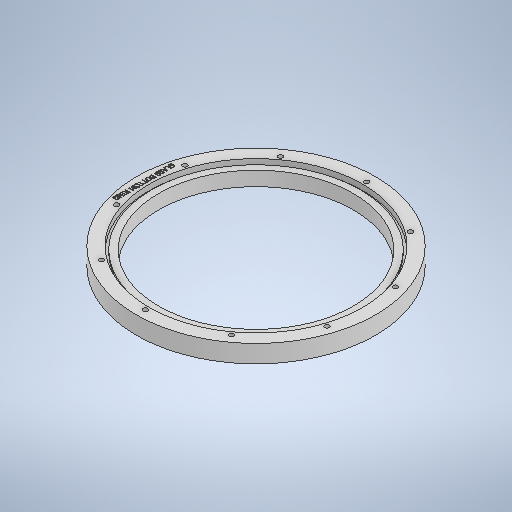
# Autodesk Inventor part: GlassBottomRing
Saved by Autodesk Inventor 2025 (Build 290162000, 162)
## iProperties
Created: 2025-06-19
Part Number: GlassBottomRing
Material: Generic
Document SubType Name: Modeling
Designer: mumin
Density: 1 g/cm^3
Appearance: Default
Author: mumin
Autodesk Inventor part; units mm, degrees
ref_plane "YZ Plane" through (0, 0, 0) normal (1, 0, 0) x (0, 1, 0)
ref_plane "XZ Plane" through (0, 0, 0) normal (0, 1, 0) x (-1, 0, 0)
ref_plane "XY Plane" through (0, 0, 0) normal (0, 0, 1) x (1, 0, 0)
sketch "Sketch1" plane through (0, 0, 0) normal (0, 1, 0) x (-1, 0, 0)
  circle A0 centre (0, 0) radius 110
  circle A1 centre (0, 0) radius 135
  dimension "d0" = 220
  dimension "d1" = 270
  constraints: 2 centre point, 2 coincident
  measures "d0" diameter of A0
  measures "d1" diameter of A1
extrude "Ring" add sketch "Sketch1" along normal blind 20
sketch "Sketch2" plane through (0, 20, 0) normal (0, 1, 0) x (1, 0, 0)
  circle A0 centre (0, 0) radius 120.5
  dimension "d4" = 241
  constraints: 1 centre point, 1 coincident
  measures "d4" diameter of A0
extrude "Glass Seat" cut sketch "Sketch2" against normal blind 3.9
sketch "Sketch3" plane through (0, 20, 0) normal (0, 1, 0) x (1, 0, 0)
  line L0 (0, 189) -> (0, -189) projected
  point P0 (0, 0)
  point P1 (0, 125)
  dimension "d14" = 125
  constraints: 1 point on line
  measures "d14" distance of point (0, 0) point (0, 125)
hole "Holes" at (0, 20, -125) direction (0, -1, 0) diameter 5.2 end through all
pattern_circular "Circular Pattern1" count 10 over 360 about axis through (0, -10, 0) along (0, 1, 0) of "Holes"
sketch "Sketch4" plane through (0, 20, 0) normal (0, 1, 0) x (1, 0, 0)
  line L0 (-123.4008, 33.078) -> (-123.4008, -40.8071) construction
  line L1 (-123.4008, -40.8071) -> (-126.5772, -40.8071) construction
  line L2 (-126.5772, -40.8071) -> (-126.5772, 33.078) construction
  line L3 (-126.5772, 33.078) -> (-123.4008, 33.078) construction
  spline S0 degree 2 poles (-128.6034, 30.4767) (-128.6034, 31.0075) (-128.2792, 31.8868) (-127.951, 32.2028) knots 0 0 0 1 2 2 2
  spline S1 degree 2 poles (-127.951, 32.2028) (-127.6188, 32.5189) (-126.6382, 32.8552) (-126.0021, 32.8552) knots 0 0 0 1 2 2 2
  spline S2 degree 2 poles (-126.0021, 32.8552) (-125.3984, 32.8552) (-124.4421, 32.5148) (-124.1018, 32.1988) knots 0 0 0 1 2 2 2
  spline S3 degree 2 poles (-124.1018, 32.1988) (-123.7736, 31.8949) (-123.417, 31.0035) (-123.417, 30.4727) knots 0 0 0 1 2 2 2
  spline S4 degree 2 poles (-123.417, 30.4727) (-123.417, 30.2174) (-123.4899, 29.7555) (-123.5548, 29.5448) knots 0 0 0 1 2 2 2
  spline S5 degree 2 poles (-123.5548, 29.5448) (-123.6034, 29.3746) (-123.7817, 28.9613) (-123.8465, 28.8357) knots 0 0 0 1 2 2 2
  line L4 (-123.8465, 28.8357) -> (-124.6488, 28.8357)
  line L5 (-124.6488, 28.8357) -> (-124.6488, 28.8925)
  spline S6 degree 2 poles (-124.6488, 28.8925) (-124.5394, 29.0181) (-124.3408, 29.2814) (-124.2274, 29.5245) knots 0 0 0 1 2 2 2
  spline S7 degree 2 poles (-124.2274, 29.5245) (-124.1261, 29.7271) (-123.9924, 30.2498) (-123.9924, 30.5497) knots 0 0 0 1 2 2 2
  spline S8 degree 2 poles (-123.9924, 30.5497) (-123.9924, 31.2709) (-125.0783, 32.1623) (-125.9818, 32.1623) knots 0 0 0 1 2 2 2
  spline S9 degree 2 poles (-125.9818, 32.1623) (-126.4843, 32.1623) (-127.2379, 31.9273) (-127.4972, 31.7044) knots 0 0 0 1 2 2 2
  spline S10 degree 2 poles (-127.4972, 31.7044) (-127.7566, 31.4897) (-128.028, 30.8819) (-128.028, 30.501) knots 0 0 0 1 2 2 2
  spline S11 degree 2 poles (-128.028, 30.501) (-128.028, 30.2215) (-127.947, 29.6623) (-127.866, 29.4719) knots 0 0 0 1 2 2 2
  line L6 (-127.866, 29.4719) -> (-126.5734, 29.4719)
  line L7 (-126.5734, 29.4719) -> (-126.5734, 30.6307)
  line L8 (-126.5734, 30.6307) -> (-125.9899, 30.6307)
  line L9 (-125.9899, 30.6307) -> (-125.9899, 28.8155)
  line L10 (-125.9899, 28.8155) -> (-128.1739, 28.8155)
  spline S12 degree 2 poles (-128.1739, 28.8155) (-128.2306, 28.9411) (-128.4048, 29.3706) (-128.4575, 29.5529) knots 0 0 0 1 2 2 2
  spline S13 degree 2 poles (-128.4575, 29.5529) (-128.5305, 29.8001) (-128.6034, 30.1972) (-128.6034, 30.4767) knots 0 0 0 1 2 2 2
  line L11 (-128.5061, 25.0837) -> (-128.5061, 27.9808)
  line L12 (-128.5061, 27.9808) -> (-123.5061, 27.9808)
  line L13 (-123.5061, 27.9808) -> (-123.5061, 27.3163)
  line L14 (-123.5061, 27.3163) -> (-127.9146, 27.3163)
  line L15 (-127.9146, 27.3163) -> (-127.9146, 25.0837)
  line L16 (-127.9146, 25.0837) -> (-128.5061, 25.0837)
  line L17 (-128.5061, 25.0999) -> (-123.5061, 23.4143)
  line L18 (-123.5061, 23.4143) -> (-123.5061, 22.5959)
  line L19 (-123.5061, 22.5959) -> (-128.5061, 20.9103)
  line L20 (-128.5061, 20.9103) -> (-128.5061, 21.6113)
  line L21 (-128.5061, 21.6113) -> (-127.1083, 22.0651)
  line L22 (-127.1083, 22.0651) -> (-127.1083, 23.9735)
  line L23 (-127.1083, 23.9735) -> (-128.5061, 24.4273)
  line L24 (-128.5061, 24.4273) -> (-128.5061, 25.0999)
  line L25 (-126.541, 22.2474) -> (-124.1869, 23.0213)
  line L26 (-124.1869, 23.0213) -> (-126.541, 23.7912)
  line L27 (-126.541, 23.7912) -> (-126.541, 22.2474)
  spline S14 degree 2 poles (-128.5953, 19.0424) (-128.5953, 19.5853) (-128.3684, 20.3471) (-128.2063, 20.6834) knots 0 0 0 1 2 2 2
  line L28 (-128.2063, 20.6834) -> (-127.3716, 20.6834)
  line L29 (-127.3716, 20.6834) -> (-127.3716, 20.6348)
  spline S15 degree 2 poles (-127.3716, 20.6348) (-127.6796, 20.3066) (-128.0199, 19.4759) (-128.0199, 19.091) knots 0 0 0 1 2 2 2
  spline S16 degree 2 poles (-128.0199, 19.091) (-128.0199, 18.5399) (-127.5621, 17.9767) (-127.1852, 17.9767) knots 0 0 0 1 2 2 2
  spline S17 degree 2 poles (-127.1852, 17.9767) (-126.8854, 17.9767) (-126.5126, 18.2725) (-126.4194, 18.5926) knots 0 0 0 1 2 2 2
  spline S18 degree 2 poles (-126.4194, 18.5926) (-126.3546, 18.8236) (-126.2655, 19.2085) (-126.1925, 19.4962) knots 0 0 0 1 2 2 2
  spline S19 degree 2 poles (-126.1925, 19.4962) (-126.1236, 19.7555) (-125.917, 20.1647) (-125.7509, 20.3228) knots 0 0 0 1 2 2 2
  spline S20 degree 2 poles (-125.7509, 20.3228) (-125.5848, 20.4767) (-125.139, 20.6469) (-124.8473, 20.6469) knots 0 0 0 1 2 2 2
  spline S21 degree 2 poles (-124.8473, 20.6469) (-124.2395, 20.6469) (-123.417, 19.6988) (-123.417, 18.9654) knots 0 0 0 1 2 2 2
  spline S22 degree 2 poles (-123.417, 18.9654) (-123.417, 18.544) (-123.5831, 17.7985) (-123.7412, 17.4784) knots 0 0 0 1 2 2 2
  line L30 (-123.7412, 17.4784) -> (-124.5353, 17.4784)
  line L31 (-124.5353, 17.4784) -> (-124.5353, 17.527)
  spline S23 degree 2 poles (-124.5353, 17.527) (-124.3165, 17.766) (-123.9924, 18.5116) (-123.9924, 18.9208) knots 0 0 0 1 2 2 2
  spline S24 degree 2 poles (-123.9924, 18.9208) (-123.9924, 19.3827) (-124.4259, 19.954) (-124.7784, 19.954) knots 0 0 0 1 2 2 2
  spline S25 degree 2 poles (-124.7784, 19.954) (-125.0945, 19.954) (-125.4713, 19.6177) (-125.5564, 19.3017) knots 0 0 0 1 2 2 2
  spline S26 degree 2 poles (-125.5564, 19.3017) (-125.6131, 19.091) (-125.759, 18.4792) (-125.8198, 18.2766) knots 0 0 0 1 2 2 2
  spline S27 degree 2 poles (-125.8198, 18.2766) (-125.9778, 17.762) (-126.6139, 17.2839) (-127.0799, 17.2839) knots 0 0 0 1 2 2 2
  spline S28 degree 2 poles (-127.0799, 17.2839) (-127.3757, 17.2839) (-127.9429, 17.5229) (-128.1415, 17.7377) knots 0 0 0 1 2 2 2
  spline S29 degree 2 poles (-128.1415, 17.7377) (-128.3603, 17.9767) (-128.5953, 18.5845) (-128.5953, 19.0424) knots 0 0 0 1 2 2 2
  spline S30 degree 2 poles (-128.5953, 15.2134) (-128.5953, 15.7563) (-128.3684, 16.5181) (-128.2063, 16.8544) knots 0 0 0 1 2 2 2
  line L32 (-128.2063, 16.8544) -> (-127.3716, 16.8544)
  line L33 (-127.3716, 16.8544) -> (-127.3716, 16.8057)
  spline S31 degree 2 poles (-127.3716, 16.8057) (-127.6796, 16.4775) (-128.0199, 15.6469) (-128.0199, 15.262) knots 0 0 0 1 2 2 2
  spline S32 degree 2 poles (-128.0199, 15.262) (-128.0199, 14.7109) (-127.5621, 14.1477) (-127.1852, 14.1477) knots 0 0 0 1 2 2 2
  spline S33 degree 2 poles (-127.1852, 14.1477) (-126.8854, 14.1477) (-126.5126, 14.4435) (-126.4194, 14.7636) knots 0 0 0 1 2 2 2
  spline S34 degree 2 poles (-126.4194, 14.7636) (-126.3546, 14.9946) (-126.2655, 15.3795) (-126.1925, 15.6672) knots 0 0 0 1 2 2 2
  spline S35 degree 2 poles (-126.1925, 15.6672) (-126.1236, 15.9265) (-125.917, 16.3357) (-125.7509, 16.4938) knots 0 0 0 1 2 2 2
  spline S36 degree 2 poles (-125.7509, 16.4938) (-125.5848, 16.6477) (-125.139, 16.8179) (-124.8473, 16.8179) knots 0 0 0 1 2 2 2
  spline S37 degree 2 poles (-124.8473, 16.8179) (-124.2395, 16.8179) (-123.417, 15.8698) (-123.417, 15.1364) knots 0 0 0 1 2 2 2
  spline S38 degree 2 poles (-123.417, 15.1364) (-123.417, 14.715) (-123.5831, 13.9694) (-123.7412, 13.6493) knots 0 0 0 1 2 2 2
  line L34 (-123.7412, 13.6493) -> (-124.5353, 13.6493)
  line L35 (-124.5353, 13.6493) -> (-124.5353, 13.698)
  spline S39 degree 2 poles (-124.5353, 13.698) (-124.3165, 13.937) (-123.9924, 14.6826) (-123.9924, 15.0918) knots 0 0 0 1 2 2 2
  spline S40 degree 2 poles (-123.9924, 15.0918) (-123.9924, 15.5537) (-124.4259, 16.125) (-124.7784, 16.125) knots 0 0 0 1 2 2 2
  spline S41 degree 2 poles (-124.7784, 16.125) (-125.0945, 16.125) (-125.4713, 15.7887) (-125.5564, 15.4727) knots 0 0 0 1 2 2 2
  spline S42 degree 2 poles (-125.5564, 15.4727) (-125.6131, 15.262) (-125.759, 14.6502) (-125.8198, 14.4476) knots 0 0 0 1 2 2 2
  spline S43 degree 2 poles (-125.8198, 14.4476) (-125.9778, 13.933) (-126.6139, 13.4549) (-127.0799, 13.4549) knots 0 0 0 1 2 2 2
  spline S44 degree 2 poles (-127.0799, 13.4549) (-127.3757, 13.4549) (-127.9429, 13.6939) (-128.1415, 13.9087) knots 0 0 0 1 2 2 2
  spline S45 degree 2 poles (-128.1415, 13.9087) (-128.3603, 14.1477) (-128.5953, 14.7555) (-128.5953, 15.2134) knots 0 0 0 1 2 2 2
  spline S46 degree 2 poles (-126.9705, 7.2393) (-127.3433, 7.2393) (-127.9146, 7.5229) (-128.101, 7.7579) knots 0 0 0 1 2 2 2
  spline S47 degree 2 poles (-128.101, 7.7579) (-128.3198, 8.0416) (-128.5061, 8.6858) (-128.5061, 9.1963) knots 0 0 0 1 2 2 2
  line L36 (-128.5061, 9.1963) -> (-128.5061, 10.6307)
  line L37 (-128.5061, 10.6307) -> (-123.5061, 10.6307)
  line L38 (-123.5061, 10.6307) -> (-123.5061, 9.3057)
  spline S48 degree 2 poles (-123.5061, 9.3057) (-123.5061, 8.7709) (-123.575, 8.2361) (-123.7087, 7.9929) knots 0 0 0 1 2 2 2
  spline S49 degree 2 poles (-123.7087, 7.9929) (-123.8506, 7.7215) (-124.3165, 7.4743) (-124.6326, 7.4743) knots 0 0 0 1 2 2 2
  spline S50 degree 2 poles (-124.6326, 7.4743) (-124.9851, 7.4743) (-125.5442, 7.8471) (-125.7023, 8.1753) knots 0 0 0 1 2 2 2
  line L39 (-125.7023, 8.1753) -> (-125.7266, 8.1753)
  spline S51 degree 2 poles (-125.7266, 8.1753) (-125.8481, 7.7296) (-126.4924, 7.2393) (-126.9705, 7.2393) knots 0 0 0 1 2 2 2
  spline S52 degree 2 poles (-126.9989, 7.9322) (-126.7152, 7.9322) (-126.3506, 8.0942) (-126.2209, 8.3373) knots 0 0 0 1 2 2 2
  spline S53 degree 2 poles (-126.2209, 8.3373) (-126.1399, 8.4954) (-126.0912, 8.8681) (-126.0912, 9.2126) knots 0 0 0 1 2 2 2
  line L40 (-126.0912, 9.2126) -> (-126.0912, 9.9662)
  line L41 (-126.0912, 9.9662) -> (-127.9389, 9.9662)
  line L42 (-127.9389, 9.9662) -> (-127.9389, 9.4273)
  spline S54 degree 2 poles (-127.9389, 9.4273) (-127.9389, 8.9897) (-127.8578, 8.4873) (-127.7282, 8.2928) knots 0 0 0 1 2 2 2
  spline S55 degree 2 poles (-127.7282, 8.2928) (-127.5945, 8.1064) (-127.2622, 7.9322) (-126.9989, 7.9322) knots 0 0 0 1 2 2 2
  spline S56 degree 2 poles (-124.7258, 8.1672) (-124.5475, 8.1672) (-124.2801, 8.2887) (-124.2031, 8.4224) knots 0 0 0 1 2 2 2
  spline S57 degree 2 poles (-124.2031, 8.4224) (-124.1139, 8.5845) (-124.0734, 8.9775) (-124.0734, 9.3301) knots 0 0 0 1 2 2 2
  line L43 (-124.0734, 9.3301) -> (-124.0734, 9.9662)
  line L44 (-124.0734, 9.9662) -> (-125.5361, 9.9662)
  line L45 (-125.5361, 9.9662) -> (-125.5361, 9.2126)
  spline S58 degree 2 poles (-125.5361, 9.2126) (-125.5361, 8.9006) (-125.4713, 8.6048) (-125.37, 8.4467) knots 0 0 0 1 2 2 2
  spline S59 degree 2 poles (-125.37, 8.4467) (-125.2728, 8.2928) (-124.9608, 8.1672) (-124.7258, 8.1672) knots 0 0 0 1 2 2 2
  spline S60 degree 2 poles (-124.0775, 3.0416) (-124.4097, 2.7579) (-125.3822, 2.4419) (-126.0061, 2.4419) knots 0 0 0 1 2 2 2
  spline S61 degree 2 poles (-126.0061, 2.4419) (-126.6139, 2.4419) (-127.5985, 2.7498) (-127.9308, 3.0416) knots 0 0 0 1 2 2 2
  spline S62 degree 2 poles (-127.9308, 3.0416) (-128.2792, 3.3495) (-128.6115, 4.1639) (-128.6115, 4.6542) knots 0 0 0 1 2 2 2
  spline S63 degree 2 poles (-128.6115, 4.6542) (-128.6115, 5.1607) (-128.2671, 5.9711) (-127.9308, 6.2668) knots 0 0 0 1 2 2 2
  spline S64 degree 2 poles (-127.9308, 6.2668) (-127.5985, 6.5545) (-126.622, 6.8625) (-126.0061, 6.8625) knots 0 0 0 1 2 2 2
  spline S65 degree 2 poles (-126.0061, 6.8625) (-125.3781, 6.8625) (-124.4219, 6.5505) (-124.0775, 6.2628) knots 0 0 0 1 2 2 2
  spline S66 degree 2 poles (-124.0775, 6.2628) (-123.7452, 5.9711) (-123.4008, 5.1566) (-123.4008, 4.6542) knots 0 0 0 1 2 2 2
  spline S67 degree 2 poles (-123.4008, 4.6542) (-123.4008, 4.1437) (-123.7574, 3.3252) (-124.0775, 3.0416) knots 0 0 0 1 2 2 2
  spline S68 degree 2 poles (-126.0061, 3.1348) (-125.5118, 3.1348) (-124.746, 3.3495) (-124.4948, 3.544) knots 0 0 0 1 2 2 2
  spline S69 degree 2 poles (-124.4948, 3.544) (-124.2355, 3.7425) (-123.9762, 4.3017) (-123.9762, 4.6502) knots 0 0 0 1 2 2 2
  spline S70 degree 2 poles (-123.9762, 4.6502) (-123.9762, 5.0108) (-124.2274, 5.5537) (-124.4948, 5.7604) knots 0 0 0 1 2 2 2
  spline S71 degree 2 poles (-124.4948, 5.7604) (-124.7501, 5.9589) (-125.5199, 6.1696) (-126.0061, 6.1696) knots 0 0 0 1 2 2 2
  spline S72 degree 2 poles (-126.0061, 6.1696) (-126.9907, 6.1696) (-128.0361, 5.343) (-128.0361, 4.6502) knots 0 0 0 1 2 2 2
  spline S73 degree 2 poles (-128.0361, 4.6502) (-128.0361, 3.9573) (-126.9907, 3.1348) (-126.0061, 3.1348) knots 0 0 0 1 2 2 2
  line L46 (-128.5061, 0.5456) -> (-124.0977, 0.5456)
  line L47 (-124.0977, 0.5456) -> (-124.0977, 2.2231)
  line L48 (-124.0977, 2.2231) -> (-123.5061, 2.2231)
  line L49 (-123.5061, 2.2231) -> (-123.5061, -1.7964)
  line L50 (-123.5061, -1.7964) -> (-124.0977, -1.7964)
  line L51 (-124.0977, -1.7964) -> (-124.0977, -0.1189)
  line L52 (-124.0977, -0.1189) -> (-128.5061, -0.1189)
  line L53 (-128.5061, -0.1189) -> (-128.5061, 0.5456)
  line L54 (-128.5061, -3.4698) -> (-124.0977, -3.4698)
  line L55 (-124.0977, -3.4698) -> (-124.0977, -1.7923)
  line L56 (-124.0977, -1.7923) -> (-123.5061, -1.7923)
  line L57 (-123.5061, -1.7923) -> (-123.5061, -5.8118)
  line L58 (-123.5061, -5.8118) -> (-124.0977, -5.8118)
  line L59 (-124.0977, -5.8118) -> (-124.0977, -4.1343)
  line L60 (-124.0977, -4.1343) -> (-128.5061, -4.1343)
  line L61 (-128.5061, -4.1343) -> (-128.5061, -3.4698)
  spline S74 degree 2 poles (-124.0775, -9.8555) (-124.4097, -10.1392) (-125.3822, -10.4552) (-126.0061, -10.4552) knots 0 0 0 1 2 2 2
  spline S75 degree 2 poles (-126.0061, -10.4552) (-126.6139, -10.4552) (-127.5985, -10.1473) (-127.9308, -9.8555) knots 0 0 0 1 2 2 2
  spline S76 degree 2 poles (-127.9308, -9.8555) (-128.2792, -9.5476) (-128.6115, -8.7332) (-128.6115, -8.2429) knots 0 0 0 1 2 2 2
  spline S77 degree 2 poles (-128.6115, -8.2429) (-128.6115, -7.7364) (-128.2671, -6.926) (-127.9308, -6.6302) knots 0 0 0 1 2 2 2
  spline S78 degree 2 poles (-127.9308, -6.6302) (-127.5985, -6.3426) (-126.622, -6.0346) (-126.0061, -6.0346) knots 0 0 0 1 2 2 2
  spline S79 degree 2 poles (-126.0061, -6.0346) (-125.3781, -6.0346) (-124.4219, -6.3466) (-124.0775, -6.6343) knots 0 0 0 1 2 2 2
  spline S80 degree 2 poles (-124.0775, -6.6343) (-123.7452, -6.926) (-123.4008, -7.7404) (-123.4008, -8.2429) knots 0 0 0 1 2 2 2
  spline S81 degree 2 poles (-123.4008, -8.2429) (-123.4008, -8.7534) (-123.7574, -9.5719) (-124.0775, -9.8555) knots 0 0 0 1 2 2 2
  spline S82 degree 2 poles (-126.0061, -9.7623) (-125.5118, -9.7623) (-124.746, -9.5476) (-124.4948, -9.3531) knots 0 0 0 1 2 2 2
  spline S83 degree 2 poles (-124.4948, -9.3531) (-124.2355, -9.1545) (-123.9762, -8.5954) (-123.9762, -8.2469) knots 0 0 0 1 2 2 2
  spline S84 degree 2 poles (-123.9762, -8.2469) (-123.9762, -7.8863) (-124.2274, -7.3434) (-124.4948, -7.1367) knots 0 0 0 1 2 2 2
  spline S85 degree 2 poles (-124.4948, -7.1367) (-124.7501, -6.9382) (-125.5199, -6.7275) (-126.0061, -6.7275) knots 0 0 0 1 2 2 2
  spline S86 degree 2 poles (-126.0061, -6.7275) (-126.9907, -6.7275) (-128.0361, -7.5541) (-128.0361, -8.2469) knots 0 0 0 1 2 2 2
  spline S87 degree 2 poles (-128.0361, -8.2469) (-128.0361, -8.9398) (-126.9907, -9.7623) (-126.0061, -9.7623) knots 0 0 0 1 2 2 2
  line L62 (-128.5061, -15.4714) -> (-128.5061, -14.8069)
  line L63 (-128.5061, -14.8069) -> (-124.199, -14.8069)
  line L64 (-124.199, -14.8069) -> (-127.1285, -13.5022)
  line L65 (-127.1285, -13.5022) -> (-127.1285, -13.097)
  line L66 (-127.1285, -13.097) -> (-124.199, -11.8045)
  line L67 (-124.199, -11.8045) -> (-128.5061, -11.8045)
  line L68 (-128.5061, -11.8045) -> (-128.5061, -11.1845)
  line L69 (-128.5061, -11.1845) -> (-123.5061, -11.1845)
  line L70 (-123.5061, -11.1845) -> (-123.5061, -12.0921)
  line L71 (-123.5061, -12.0921) -> (-126.2898, -13.3401)
  line L72 (-126.2898, -13.3401) -> (-123.5061, -14.5476)
  line L73 (-123.5061, -14.5476) -> (-123.5061, -15.4714)
  line L74 (-123.5061, -15.4714) -> (-128.5061, -15.4714)
  line L75 (-128.5061, -22.5014) -> (-128.5061, -21.6383)
  line L76 (-128.5061, -21.6383) -> (-126.5167, -20.0581)
  line L77 (-126.5167, -20.0581) -> (-126.5167, -19.2964)
  line L78 (-126.5167, -19.2964) -> (-128.5061, -19.2964)
  line L79 (-128.5061, -19.2964) -> (-128.5061, -18.6319)
  line L80 (-128.5061, -18.6319) -> (-123.5061, -18.6319)
  line L81 (-123.5061, -18.6319) -> (-123.5061, -19.9203)
  spline S88 degree 2 poles (-123.5061, -19.9203) (-123.5061, -20.3498) (-123.5993, -20.9293) (-123.7695, -21.1926) knots 0 0 0 1 2 2 2
  spline S89 degree 2 poles (-123.7695, -21.1926) (-123.9397, -21.456) (-124.4705, -21.7599) (-124.8635, -21.7599) knots 0 0 0 1 2 2 2
  spline S90 degree 2 poles (-124.8635, -21.7599) (-125.4105, -21.7599) (-126.152, -21.2007) (-126.3303, -20.7226) knots 0 0 0 1 2 2 2
  line L82 (-126.3303, -20.7226) -> (-128.5061, -22.5014)
  spline S91 degree 2 poles (-124.9162, -21.067) (-124.6974, -21.067) (-124.3611, -20.9131) (-124.2517, -20.751) knots 0 0 0 1 2 2 2
  spline S92 degree 2 poles (-124.2517, -20.751) (-124.1585, -20.6092) (-124.0815, -20.2323) (-124.0815, -19.9568) knots 0 0 0 1 2 2 2
  line L83 (-124.0815, -19.9568) -> (-124.0815, -19.2964)
  line L84 (-124.0815, -19.2964) -> (-125.9616, -19.2964)
  line L85 (-125.9616, -19.2964) -> (-125.9616, -19.8798)
  spline S93 degree 2 poles (-125.9616, -19.8798) (-125.9616, -20.1675) (-125.8603, -20.6254) (-125.7023, -20.7834) knots 0 0 0 1 2 2 2
  spline S94 degree 2 poles (-125.7023, -20.7834) (-125.5645, -20.9293) (-125.1755, -21.067) (-124.9162, -21.067) knots 0 0 0 1 2 2 2
  line L86 (-128.5061, -24.6408) -> (-128.5061, -22.704)
  line L87 (-128.5061, -22.704) -> (-127.9956, -22.704)
  line L88 (-127.9956, -22.704) -> (-127.9956, -23.3401)
  line L89 (-127.9956, -23.3401) -> (-124.0167, -23.3401)
  line L90 (-124.0167, -23.3401) -> (-124.0167, -22.704)
  line L91 (-124.0167, -22.704) -> (-123.5061, -22.704)
  line L92 (-123.5061, -22.704) -> (-123.5061, -24.6408)
  line L93 (-123.5061, -24.6408) -> (-124.0167, -24.6408)
  line L94 (-124.0167, -24.6408) -> (-124.0167, -24.0046)
  line L95 (-124.0167, -24.0046) -> (-127.9956, -24.0046)
  line L96 (-127.9956, -24.0046) -> (-127.9956, -24.6408)
  line L97 (-127.9956, -24.6408) -> (-128.5061, -24.6408)
  line L98 (-128.5061, -29.0411) -> (-128.5061, -28.2956)
  line L99 (-128.5061, -28.2956) -> (-124.195, -26.0832)
  line L100 (-124.195, -26.0832) -> (-128.5061, -26.0832)
  line L101 (-128.5061, -26.0832) -> (-128.5061, -25.4633)
  line L102 (-128.5061, -25.4633) -> (-123.5061, -25.4633)
  line L103 (-123.5061, -25.4633) -> (-123.5061, -26.4074)
  line L104 (-123.5061, -26.4074) -> (-127.4648, -28.4212)
  line L105 (-127.4648, -28.4212) -> (-123.5061, -28.4212)
  line L106 (-123.5061, -28.4212) -> (-123.5061, -29.0411)
  line L107 (-123.5061, -29.0411) -> (-128.5061, -29.0411)
  spline S95 degree 2 poles (-128.6034, -32.1489) (-128.6034, -31.6181) (-128.2792, -30.7388) (-127.951, -30.4228) knots 0 0 0 1 2 2 2
  spline S96 degree 2 poles (-127.951, -30.4228) (-127.6188, -30.1067) (-126.6382, -29.7704) (-126.0021, -29.7704) knots 0 0 0 1 2 2 2
  spline S97 degree 2 poles (-126.0021, -29.7704) (-125.3984, -29.7704) (-124.4421, -30.1108) (-124.1018, -30.4268) knots 0 0 0 1 2 2 2
  spline S98 degree 2 poles (-124.1018, -30.4268) (-123.7736, -30.7307) (-123.417, -31.6221) (-123.417, -32.1529) knots 0 0 0 1 2 2 2
  spline S99 degree 2 poles (-123.417, -32.1529) (-123.417, -32.4082) (-123.4899, -32.8701) (-123.5548, -33.0808) knots 0 0 0 1 2 2 2
  spline S100 degree 2 poles (-123.5548, -33.0808) (-123.6034, -33.251) (-123.7817, -33.6643) (-123.8465, -33.7899) knots 0 0 0 1 2 2 2
  line L108 (-123.8465, -33.7899) -> (-124.6488, -33.7899)
  line L109 (-124.6488, -33.7899) -> (-124.6488, -33.7332)
  spline S101 degree 2 poles (-124.6488, -33.7332) (-124.5394, -33.6075) (-124.3408, -33.3442) (-124.2274, -33.1011) knots 0 0 0 1 2 2 2
  spline S102 degree 2 poles (-124.2274, -33.1011) (-124.1261, -32.8985) (-123.9924, -32.3758) (-123.9924, -32.0759) knots 0 0 0 1 2 2 2
  spline S103 degree 2 poles (-123.9924, -32.0759) (-123.9924, -31.3547) (-125.0783, -30.4633) (-125.9818, -30.4633) knots 0 0 0 1 2 2 2
  spline S104 degree 2 poles (-125.9818, -30.4633) (-126.4843, -30.4633) (-127.2379, -30.6983) (-127.4972, -30.9212) knots 0 0 0 1 2 2 2
  spline S105 degree 2 poles (-127.4972, -30.9212) (-127.7566, -31.1359) (-128.028, -31.7437) (-128.028, -32.1246) knots 0 0 0 1 2 2 2
  spline S106 degree 2 poles (-128.028, -32.1246) (-128.028, -32.4041) (-127.947, -32.9633) (-127.866, -33.1537) knots 0 0 0 1 2 2 2
  line L110 (-127.866, -33.1537) -> (-126.5734, -33.1537)
  line L111 (-126.5734, -33.1537) -> (-126.5734, -31.9949)
  line L112 (-126.5734, -31.9949) -> (-125.9899, -31.9949)
  line L113 (-125.9899, -31.9949) -> (-125.9899, -33.8101)
  line L114 (-125.9899, -33.8101) -> (-128.1739, -33.8101)
  spline S107 degree 2 poles (-128.1739, -33.8101) (-128.2306, -33.6845) (-128.4048, -33.255) (-128.4575, -33.0727) knots 0 0 0 1 2 2 2
  spline S108 degree 2 poles (-128.4575, -33.0727) (-128.5305, -32.8255) (-128.6034, -32.4285) (-128.6034, -32.1489) knots 0 0 0 1 2 2 2
  point P0 (0, 0)
  constraints: 2 other
emboss "Emboss1" sketch "Sketch4" operation cut depth 1 direction (0, -1, 0)
sketch "Sketch5" plane through (0, 16.1, 0) normal (0, 1, 0) x (1, 0, 0)
  circle A0 centre (0, 0) radius 120.5
  circle A1 centre (0, 0) radius 117.5
  dimension "d21" = 241
  dimension "d22" = 3
  constraints: 2 centre point, 2 coincident
  measures "d21" diameter of A0
  measures "d22" radial gap between concentric circles of A0 A1
extrude "Extrusion3" cut sketch "Sketch5" against normal blind 2.5
body "Solid1"
